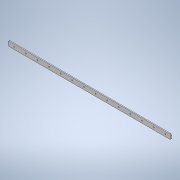
# Autodesk Inventor part: Linear Rail Screw Plate
Saved by Autodesk Inventor 2022 (Build 260153000, 153)
## iProperties
Created: 2022-03-21
Part Number: Linear Rail Screw Plate
Material: Generic
Document SubType Name: Modeling
Designer: Nick
Density: 1 g/cm^3
Appearance: Default
Author: Nick
Autodesk Inventor part; units mm, degrees
ref_plane "YZ Plane" through (0, 0, 0) normal (1, 0, 0) x (0, 1, 0)
ref_plane "XZ Plane" through (0, 0, 0) normal (0, 1, 0) x (-1, 0, 0)
ref_plane "XY Plane" through (0, 0, 0) normal (0, 0, 1) x (1, 0, 0)
sketch "Sketch1" plane through (0, 0, 0) normal (0, 0, 1) x (1, 0, 0)
  line L0 (0, 0) -> (350, 0)
  line L1 (350, 0) -> (350, 10)
  line L2 (350, 10) -> (0, 10)
  line L3 (0, 10) -> (0, 0)
  dimension "d0" = 350
  dimension "d1" = 10
  constraints: 8 end point, 2 parallel, 1 horizontal, 1 perpendicular
  measures "d0" distance of L2.end L1.end
  measures "d1" distance of L1.end L0.end
extrude "Extrusion1" add sketch "Sketch1" along normal blind 2
sketch "Sketch2" plane through (0, 0, 2) normal (0, 0, 1) x (1, 0, 0)
  line L0 (0, 10) -> (0, 0) projected
  point P0 (13, 5)
  point P1 (0, 5)
  dimension "d4" = 13
  constraints: 1 horizontal alignment, 1 midpoint
  measures "d4" distance from line of point (13, 5) L0
hole "Hole1" at (13, 5, 2) direction (0, 0, -1) diameter 2.459 end through all thread size "M3x0.5" class "6H" standard "ANSI Metric M Profile"
pattern_linear "Rectangular Pattern1" count 14 spacing 25 along (1, 0, 0) of "Hole1"
fillet "Fillet1" radius 2 4 edges at (0, 0, 1) (0, 10, 1) (350, 0, 1) (350, 10, 1)
body "Solid1"
